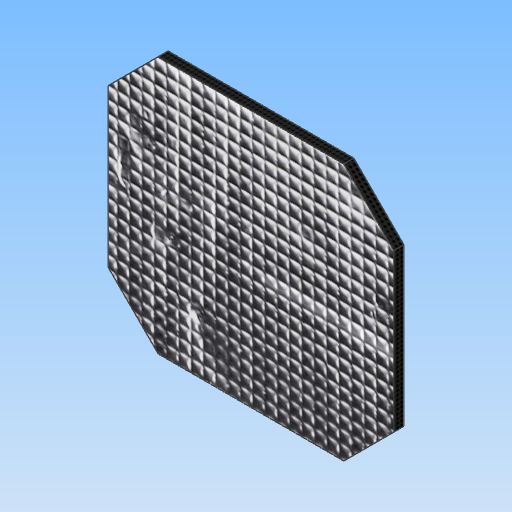
# Autodesk Inventor part: утепление стола
Saved by Autodesk Inventor 2017 (Build 210142000, 142)
## iProperties
Part Number: утепление стола
Material: Типовые
Document SubType Name: Modeling
Designer: Max
Mass: 234.85 g
Surface Area: 718.459 cm^2
Volume: 234.85 cm^3
Density: 1 g/cm^3
Appearance: Пластина башмака
Author: Max
Autodesk Inventor part; units mm, degrees
ref_plane "YZ Plane" through (0, 0, 0) normal (1, 0, 0) x (0, 1, 0)
ref_plane "XZ Plane" through (0, 0, 0) normal (0, 1, 0) x (-1, 0, 0)
ref_plane "XY Plane" through (0, 0, 0) normal (0, 0, 1) x (1, 0, 0)
sketch "Эскиз1" plane through (0, 0, 0) normal (0, 0, 1) x (1, 0, 0)
  line L0 (11.0194, 105.4233) -> (11.0194, 99.2429)
  line L1 (11.0194, 99.2429) -> (-11.0194, 99.2429)
  line L2 (-11.0194, 99.2429) -> (-11.0194, 105.4233)
  line L3 (-11.0194, 105.4233) -> (11.0194, 105.4233)
  circle A0 centre (104, 76) radius 1.481
  circle A1 centre (104, -76) radius 1.481
  circle A2 centre (-104, -76) radius 1.481
  circle A3 centre (-104, 76) radius 1.481
  arc A4 (135.5, -107) -> (137.5, -105) centre (135.5, -105) ccw
  line L4 (137.5, 105) -> (137.5, -105)
  arc A5 (137.5, 105) -> (135.5, 107) centre (135.5, 105) ccw
  line L5 (-135.5, 107) -> (135.5, 107)
  arc A6 (-135.5, 107) -> (-137.5, 105) centre (-135.5, 105) ccw
  line L6 (-137.5, -105) -> (-137.5, 105)
  arc A7 (-137.5, -105) -> (-135.5, -107) centre (-135.5, -105) ccw
  line L7 (135.5, -107) -> (-135.5, -107)
  line L8 (-132.5, -102) -> (-132.5, 102)
  line L9 (-132.5, 102) -> (132.5, 102)
  line L10 (132.5, 102) -> (132.5, -102)
  line L11 (132.5, -102) -> (-132.5, -102)
  point P0 (0, 0)
  dimension "d0" = 5
  constraints: 24 end point, 8 centre point, 8 point on circle, 3 other
  measures "d0" distance between parallel lines of L7 L11
extrude "Выдавливание1" add sketch "Эскиз1" along normal blind 7 contours L9 L10 L11 L8 L2 L1 L0 | L0 L1 L2 L9
sketch "Эскиз2" plane through (0, 0, 7) normal (0, 0, 1) x (1, 0, 0)
  line L0 (-146.9193, 158.9761) -> (149.0915, 158.9761) construction
  line L1 (149.0915, 158.9761) -> (149.0915, -137.0348) construction
  line L2 (149.0915, -137.0348) -> (-146.9193, -137.0348) construction
  line L3 (-146.9193, -137.0348) -> (-146.9193, 158.9761) construction
  point P0 (0, 0)
  constraints: 2 other
decal "Маркировка1"
sketch "Эскиз4" plane through (0, 0, 0) normal (0, 0, -1) x (-1, 0, 0)
  line L0 (-100, 90) -> (100, 90)
  line L1 (100, 90) -> (100, -90)
  line L2 (100, -90) -> (-100, -90)
  line L3 (-100, -90) -> (-100, 90)
  line L4 (-100, 90) -> (100, -90) construction
  line L5 (100, 90) -> (-100, -90) construction
  line L6 (100, -55) -> (65, -90)
  line L7 (-65, -90) -> (-100, -55)
  line L8 (-100, 55) -> (-65, 90)
  line L9 (100, 55) -> (65, 90)
  line L10 (-65, 90) -> (65, 90) construction
  line L11 (65, 90) -> (65, -90) construction
  line L12 (65, -90) -> (-65, -90) construction
  line L13 (-65, -90) -> (-65, 90) construction
  line L14 (-65, 90) -> (65, -90) construction
  line L15 (65, 90) -> (-65, -90) construction
  line L16 (-276.1466, 193.443) -> (276.1466, 193.443)
  line L17 (276.1466, 193.443) -> (276.1466, -193.443)
  line L18 (276.1466, -193.443) -> (-276.1466, -193.443)
  line L19 (-276.1466, -193.443) -> (-276.1466, 193.443)
  line L20 (-276.1466, 193.443) -> (276.1466, -193.443) construction
  line L21 (276.1466, 193.443) -> (-276.1466, -193.443) construction
  point P0 (0, 0)
  point P1 (0, 0)
  dimension "d18" = 200
  dimension "d19" = 180
  dimension "d20" = 45
  dimension "d21" = 45
  dimension "d22" = 45
  dimension "d23" = 45
  dimension "d24" = 130
  constraints: 44 end point, 8 midpoint, 8 point on line, 6 parallel, 4 perpendicular, 3 horizontal
  measures "d18" distance of L1.end L2.end
  measures "d19" distance of L0.end L1.end
  measures "d20" angle of L1 L6
  measures "d21" angle of L7 L2
  measures "d22" angle of L3 L8
  measures "d23" angle of L0 L9
  measures "d24" distance of L7.start L6.end
extrude "Выдавливание3" cut sketch "Эскиз4" against normal blind 10 contours L0 L8 L3 | L0 L1 L9 | L7 L2 L3 | L1 L2 L6 | L16 L17 L18 L19
